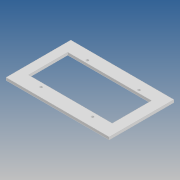
# Autodesk Inventor part: KB33-046-004-004 - Центральная верхняя пластина
Saved by Autodesk Inventor 2020 (Build 240168000, 168)
## iProperties
Created: 2021-06-25
Part Number: KB33-046-004-004 - Центральная верхняя пластина
Material: Типовые
Document SubType Name: Modeling
Designer: Петров Иван
Mass: 32.364 g
Surface Area: 199.792 cm^2
Volume: 32.364 cm^3
Density: 1 g/cm^3
Appearance: По умолчанию
Author: Петров Иван
Autodesk Inventor part; units mm, degrees
ref_plane "YZ Plane" through (0, 0, 0) normal (1, 0, 0) x (0, 1, 0)
ref_plane "XZ Plane" through (0, 0, 0) normal (0, 1, 0) x (-1, 0, 0)
ref_plane "XY Plane" through (0, 0, 0) normal (0, 0, 1) x (1, 0, 0)
sketch "Эскиз2" plane through (-80, 0, -49.5) normal (0, 1, 0) x (-1, 0, 0)
  circle A0 centre (-40, 85.5) radius 1.85
  circle A1 centre (-40, 13.5) radius 1.85
  circle A2 centre (-120, 85.5) radius 1.85
  circle A3 centre (-120, 13.5) radius 1.85
  line L0 (0, 99) -> (0, 68.3189)
  line L1 (0, 99) -> (-160, 99)
  line L2 (-160, 0) -> (0, 0)
  line L3 (-160, 30.6811) -> (-160, 0)
  line L4 (0, 99) -> (-160, 99)
  line L5 (-160, 99) -> (-160, 0)
  line L6 (-160, 0) -> (0, 0)
  line L7 (0, 0) -> (0, 99)
  line L8 (-14, 79) -> (-144, 79)
  line L9 (-144, 79) -> (-144, 18)
  line L10 (-144, 18) -> (-14, 18)
  line L11 (-14, 18) -> (-14, 79)
  dimension "d9" = 130
  dimension "d10" = 61
  dimension "d11" = 16
  dimension "d12" = 20
  constraints: 24 end point, 4 centre point, 4 horizontal, 4 parallel, 3 vertical, 2 perpendicular, 4 other
  measures "d9" distance of L10.end L9.end
  measures "d10" distance of L9.end L8.end
  measures "d11" distance between parallel lines of L5 L9
  measures "d12" distance between parallel lines of L4 L8
extrude "Выдавливание2" add sketch "Эскиз2" along normal blind 4
thicken "Толщина1" operation add thickness 0.7 both sides no extend neighbours yes toward (0, 0, 1) faces at (-26.6667, 1.3333, 49.5)
thicken "Толщина2" operation add thickness 0.7 both sides no extend neighbours yes toward (0, 0, -1) faces at (26.6667, 1.3333, -49.5)
